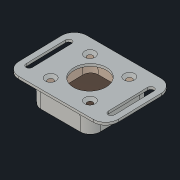
# Autodesk Inventor part: sliderr
Saved by Autodesk Inventor 2022 (Build 260153000, 153)
## iProperties
Created: 2021-12-03
Part Number: sliderr
Material: Generic
Document SubType Name: Modeling
Designer: alber
Density: 1 g/cm^3
Appearance: Default
Author: alber
Autodesk Inventor part; units mm, degrees
ref_plane "YZ Plane" through (0, 0, 0) normal (1, 0, 0) x (0, 1, 0)
ref_plane "XZ Plane" through (0, 0, 0) normal (0, 1, 0) x (-1, 0, 0)
ref_plane "XY Plane" through (0, 0, 0) normal (0, 0, 1) x (1, 0, 0)
ref_plane "Work Plane1" through (4.8385, 19.1943, 116.7457) normal (0, 0.9997114, 0.0240226) x (0, 0.0240226, -0.9997114)
sketch "Sketch1" plane through (4.8385, 19.1943, 116.7457) normal (0, 0.9997114, 0.0240226) x (0, 0.0240226, -0.9997114)
  line L0 (-15.5, 20.3) -> (15.5, 20.3) projected
  arc A0 (-15.5, 20.3) -> (-20.3, 15.5) centre (-15.5, 15.5) ccw projected
  line L1 (-20.3, -15.5) -> (-20.3, 15.5) projected
  arc A1 (-20.3, -15.5) -> (-15.5, -20.3) centre (-15.5, -15.5) ccw projected
  line L2 (15.5, -20.3) -> (-15.5, -20.3) projected
  arc A2 (15.5, -20.3) -> (20.3, -15.5) centre (15.5, -15.5) ccw projected
  line L3 (20.3, 15.5) -> (20.3, -15.5) projected
  arc A3 (20.3, 15.5) -> (15.5, 20.3) centre (15.5, 15.5) ccw projected
  circle A4 centre (-15.5, -15.5) radius 2.2 projected
  circle A5 centre (-15.5, 15.5) radius 2.2 projected
  circle A6 centre (0, 0) radius 11 projected
  circle A7 centre (15.5, -15.5) radius 2.2 projected
  circle A8 centre (15.5, 15.5) radius 2.2 projected
  circle A9 centre (0, 0) radius 13
  line L4 (-80.9362, 34.8457) -> (36.4047, 34.8457)
  line L5 (14.4725, 29.7685) -> (-11.5275, 29.7685)
  line L6 (14.4725, -29.9228) -> (-11.5275, -29.9228)
  line L7 (-80.9362, -35) -> (36.4047, -35)
  line L8 (-12.1439, 29.8457) -> (-80.9362, 29.8457)
  line L9 (-75.5135, 25.4228) -> (37.0415, 25.4228)
  line L10 (-75.5135, -25.5772) -> (37.0415, -25.5772)
  line L11 (-26.724, 15.5) -> (-26.724, -15.5)
  arc A10 (-20.4426, -25.5772) -> (-20.3, -25.6459) centre (-15.5, -15.5) ccw
  line L12 (26.724, -15.5) -> (26.724, 15.5)
  line L13 (-15.5, 29.8457) -> (15.5, 29.8457)
  line L14 (15.5, 34.8457) -> (-15.5, 34.8457)
  circle A11 centre (-15.5, 32.3457) radius 2.5
  circle A12 centre (15.5, 32.3457) radius 2.5
  line L15 (37.0415, 39.2685) -> (-115.5135, 39.2685)
  line L16 (-20.3, 15.5) -> (-17.7, 15.5)
  line L17 (26.724, 15.5) -> (26.724, 29.2685)
  line L18 (16.724, 39.2685) -> (-16.724, 39.2685)
  line L19 (-26.724, 29.2685) -> (-26.724, 15.5)
  arc A13 (-16.724, 39.2685) -> (-26.724, 29.2685) centre (-16.724, 29.2685) ccw
  arc A14 (26.724, 29.2685) -> (16.724, 39.2685) centre (16.724, 29.2685) ccw
  line L20 (-26.724, 0) -> (26.724, 0)
  line L21 (14.4725, -29.7685) -> (-11.5275, -29.7685)
  line L22 (-15.5, -29.8457) -> (15.5, -29.8457)
  line L23 (15.5, -34.8457) -> (-15.5, -34.8457)
  circle A15 centre (-15.5, -32.3457) radius 2.5
  circle A16 centre (15.5, -32.3457) radius 2.5
  line L24 (26.724, -15.5) -> (26.724, -29.2685)
  line L25 (16.724, -39.2685) -> (-16.724, -39.2685)
  line L26 (-26.724, -29.2685) -> (-26.724, -15.5)
  arc A17 (-26.724, -29.2685) -> (-16.724, -39.2685) centre (-16.724, -29.2685) ccw
  arc A18 (16.724, -39.2685) -> (26.724, -29.2685) centre (16.724, -29.2685) ccw
  point P0 (116.2509, 4.8385)
  point P1 (26.724, 39.2685)
  point P2 (36.4047, -34.8457)
  point P3 (-12.1439, -29.8457)
  point P4 (37.0415, -25.4228)
  point P5 (37.0415, -39.2685)
  point P6 (26.724, -39.2685)
  point P7 (26.724, -15.5)
  point P8 (16.724, 39.2685)
  point P9 (-16.724, 39.2685)
  point P10 (-15.5, -34.8457)
  point P11 (-15.5, -29.8457)
  point P12 (-15.5, 34.8457)
  point P13 (15.5, 34.8457)
  point P14 (15.5, 29.8457)
  point P15 (-15.5, 29.8457)
  dimension "d0" = 2
  dimension "d16" = 5.1228
  dimension "d17" = 5
  dimension "d18" = 5
  dimension "d19" = 10
  constraints: 46 end point, 20 symmetric about line, 10 centre point, 10 horizontal, 10 point on circle, 10 point on line, 4 tangent, 3 parallel, 2 midpoint, 1 collinear, 1 equal radius, 1 horizontal alignment, 1 perpendicular, 21 other
  measures "d0" radial gap between concentric circles of A6 A9
  measures "d16" distance between parallel lines of L9 L0
  measures "d17" diameter of A11
  measures "d18" diameter of A12
  measures "d19" radius of A13
extrude "Extrusion1" add sketch "Sketch1" along normal blind 2 contours A0 L1 L20 L11 L19 L9 L17 L12 L3 A3 L0 | L0 A3 L3 L20 A9 L1 A0 | L20 A9 L3 A2 L2 A1 L1 | L1 A1 L2 A2 L3 L20 L12 L24 L10 L26 L11 | L19 A13 L8 L13 A12 L4 A14 L17 L9 | L10 L24 A18 L7 A17 L26 | A13 L4 A11 L8 | L7 A18 L25 A17 | L4 A13 L15 A14
sketch "Sketch2" plane through (4.8385, 19.1943, 116.7457) normal (0, -0.9997114, -0.0240226) x (1, 0, 0)
  line L0 (-20.5, -15.5) -> (-20.5, 15.5) projected
  arc A0 (-20.5, -15.5) -> (-15.5, -20.5) centre (-15.5, -15.5) ccw projected
  line L1 (15.5, -20.5) -> (-15.5, -20.5) projected
  arc A1 (15.5, -20.5) -> (20.5, -15.5) centre (15.5, -15.5) ccw projected
  line L2 (20.5, 15.5) -> (20.5, -15.5) projected
  arc A2 (20.5, 15.5) -> (15.5, 20.5) centre (15.5, 15.5) ccw projected
  line L3 (-15.5, 20.5) -> (15.5, 20.5) projected
  arc A3 (-15.5, 20.5) -> (-20.5, 15.5) centre (-15.5, 15.5) ccw projected
  circle A4 centre (0, 0) radius 4 projected
  circle A5 centre (7.248, 7.248) radius 1.45 projected
  arc A6 (-21.5, -15.5) -> (-15.5, -21.5) centre (-15.5, -15.5) ccw
  line L4 (-21.5, -15.5) -> (-21.5, 15.5)
  arc A7 (-15.5, 21.5) -> (-21.5, 15.5) centre (-15.5, 15.5) ccw
  line L5 (-15.5, 21.5) -> (15.5, 21.5)
  arc A8 (21.5, 15.5) -> (15.5, 21.5) centre (15.5, 15.5) ccw
  line L6 (21.5, 15.5) -> (21.5, -15.5)
  arc A9 (15.5, -21.5) -> (21.5, -15.5) centre (15.5, -15.5) ccw
  line L7 (15.5, -21.5) -> (-15.5, -21.5)
  arc A10 (-23.5, -15.5) -> (-15.5, -23.5) centre (-15.5, -15.5) ccw
  line L8 (-23.5, -15.5) -> (-23.5, 15.5)
  arc A11 (-15.5, 23.5) -> (-23.5, 15.5) centre (-15.5, 15.5) ccw
  line L9 (-15.5, 23.5) -> (15.5, 23.5)
  arc A12 (23.5, 15.5) -> (15.5, 23.5) centre (15.5, 15.5) ccw
  line L10 (23.5, 15.5) -> (23.5, -15.5)
  arc A13 (15.5, -23.5) -> (23.5, -15.5) centre (15.5, -15.5) ccw
  line L11 (15.5, -23.5) -> (-15.5, -23.5)
  point P0 (-4.8385, -116.2509)
  dimension "d11" = 1
  dimension "d12" = 2
  constraints: 16 end point, 16 point on circle, 8 centre point, 14 other
  measures "d11" distance between parallel lines of L1 L7
  measures "d12" distance between parallel lines of L7 L11
extrude "Extrusion2" add sketch "Sketch2" along normal blind 8.35 contours L8 A11 L9 A12 L10 A13 L11 A10
fillet "Fillet1" radius 2 8 edges at (-16.3183, 19.7025, 95.5949) (-18.6615, 19.1943, 116.7457) (-16.3183, 18.686, 137.8964) (4.8385, 18.6297, 140.2389) (25.9954, 18.686, 137.8964) (28.3385, 19.1943, 116.7457) (25.9954, 19.7025, 95.5949) (4.8385, 19.7588, 93.2524)
move faces "Move1" translate (0, -6.998, -0.1682) faces at (-0.3281, 10.3142, 138.7053)
chamfer "Chamfer1" distance 2 angle 45 4 edges at (-10.6615, 20.7685, 134.4886) (20.3385, 21.5132, 103.4975) (-10.6615, 21.5132, 103.4975) (20.3385, 20.7685, 134.4886)
body "Solid1"
